Autodesk Inventor part; units mm, degrees
(part 2 of 5)
sketch "Block3" plane through (0, 0, 0) normal (0, 0, 1) x (1, 0, 0)
  line L0 (3.025, -7.2875) -> (16.025, -7.2875)
  line L1 (3.025, -21.2875) -> (16.025, -21.2875)
  line L2 (2.525, -7.7875) -> (2.525, -20.7875)
  line L3 (16.525, -7.7875) -> (16.525, -20.7875)
  arc A0 (3.025, -7.2875) -> (2.525, -7.7875) centre (3.025, -7.7875) ccw
  arc A1 (16.525, -7.7875) -> (16.025, -7.2875) centre (16.025, -7.7875) ccw
  arc A2 (2.525, -20.7875) -> (3.025, -21.2875) centre (3.025, -20.7875) ccw
  arc A3 (16.025, -21.2875) -> (16.525, -20.7875) centre (16.025, -20.7875) ccw
  line L4 (41.125, -7.2875) -> (54.125, -7.2875)
  line L5 (41.125, -21.2875) -> (54.125, -21.2875)
  line L6 (40.625, -7.7875) -> (40.625, -20.7875)
  line L7 (54.625, -7.7875) -> (54.625, -20.7875)
  arc A4 (41.125, -7.2875) -> (40.625, -7.7875) centre (41.125, -7.7875) ccw
  arc A5 (54.625, -7.7875) -> (54.125, -7.2875) centre (54.125, -7.7875) ccw
  arc A6 (40.625, -20.7875) -> (41.125, -21.2875) centre (41.125, -20.7875) ccw
  arc A7 (54.125, -21.2875) -> (54.625, -20.7875) centre (54.125, -20.7875) ccw
  line L8 (60.175, -7.2875) -> (73.175, -7.2875)
  line L9 (60.175, -21.2875) -> (73.175, -21.2875)
  line L10 (59.675, -7.7875) -> (59.675, -20.7875)
  line L11 (73.675, -7.7875) -> (73.675, -20.7875)
  arc A8 (60.175, -7.2875) -> (59.675, -7.7875) centre (60.175, -7.7875) ccw
  arc A9 (73.675, -7.7875) -> (73.175, -7.2875) centre (73.175, -7.7875) ccw
  arc A10 (59.675, -20.7875) -> (60.175, -21.2875) centre (60.175, -20.7875) ccw
  arc A11 (73.175, -21.2875) -> (73.675, -20.7875) centre (73.175, -20.7875) ccw
  line L12 (79.225, -7.2875) -> (92.225, -7.2875)
  line L13 (79.225, -21.2875) -> (92.225, -21.2875)
  line L14 (78.725, -7.7875) -> (78.725, -20.7875)
  line L15 (92.725, -7.7875) -> (92.725, -20.7875)
  arc A12 (79.225, -7.2875) -> (78.725, -7.7875) centre (79.225, -7.7875) ccw
  arc A13 (92.725, -7.7875) -> (92.225, -7.2875) centre (92.225, -7.7875) ccw
  arc A14 (78.725, -20.7875) -> (79.225, -21.2875) centre (79.225, -20.7875) ccw
  arc A15 (92.225, -21.2875) -> (92.725, -20.7875) centre (92.225, -20.7875) ccw
  line L16 (98.275, -7.2875) -> (111.275, -7.2875)
  line L17 (98.275, -21.2875) -> (111.275, -21.2875)
  line L18 (97.775, -7.7875) -> (97.775, -20.7875)
  line L19 (111.775, -7.7875) -> (111.775, -20.7875)
  arc A16 (98.275, -7.2875) -> (97.775, -7.7875) centre (98.275, -7.7875) ccw
  arc A17 (111.775, -7.7875) -> (111.275, -7.2875) centre (111.275, -7.7875) ccw
  arc A18 (97.775, -20.7875) -> (98.275, -21.2875) centre (98.275, -20.7875) ccw
  arc A19 (111.275, -21.2875) -> (111.775, -20.7875) centre (111.275, -20.7875) ccw
  line L20 (126.85, -7.2875) -> (139.85, -7.2875)
  line L21 (126.85, -21.2875) -> (139.85, -21.2875)
  line L22 (126.35, -7.7875) -> (126.35, -20.7875)
  line L23 (140.35, -7.7875) -> (140.35, -20.7875)
  arc A20 (126.85, -7.2875) -> (126.35, -7.7875) centre (126.85, -7.7875) ccw
  arc A21 (140.35, -7.7875) -> (139.85, -7.2875) centre (139.85, -7.7875) ccw
  arc A22 (126.35, -20.7875) -> (126.85, -21.2875) centre (126.85, -20.7875) ccw
  arc A23 (139.85, -21.2875) -> (140.35, -20.7875) centre (139.85, -20.7875) ccw
  line L24 (145.9, -7.2875) -> (158.9, -7.2875)
  line L25 (145.9, -21.2875) -> (158.9, -21.2875)
  line L26 (145.4, -7.7875) -> (145.4, -20.7875)
  line L27 (159.4, -7.7875) -> (159.4, -20.7875)
  arc A24 (145.9, -7.2875) -> (145.4, -7.7875) centre (145.9, -7.7875) ccw
  arc A25 (159.4, -7.7875) -> (158.9, -7.2875) centre (158.9, -7.7875) ccw
  arc A26 (145.4, -20.7875) -> (145.9, -21.2875) centre (145.9, -20.7875) ccw
  arc A27 (158.9, -21.2875) -> (159.4, -20.7875) centre (158.9, -20.7875) ccw
  line L28 (164.95, -7.2875) -> (177.95, -7.2875)
  line L29 (164.95, -21.2875) -> (177.95, -21.2875)
  line L30 (164.45, -7.7875) -> (164.45, -20.7875)
  line L31 (178.45, -7.7875) -> (178.45, -20.7875)
  arc A28 (164.95, -7.2875) -> (164.45, -7.7875) centre (164.95, -7.7875) ccw
  arc A29 (178.45, -7.7875) -> (177.95, -7.2875) centre (177.95, -7.7875) ccw
  arc A30 (164.45, -20.7875) -> (164.95, -21.2875) centre (164.95, -20.7875) ccw
  arc A31 (177.95, -21.2875) -> (178.45, -20.7875) centre (177.95, -20.7875) ccw
  line L32 (184, -7.2875) -> (197, -7.2875)
  line L33 (184, -21.2875) -> (197, -21.2875)
  line L34 (183.5, -7.7875) -> (183.5, -20.7875)
  line L35 (197.5, -7.7875) -> (197.5, -20.7875)
  arc A32 (184, -7.2875) -> (183.5, -7.7875) centre (184, -7.7875) ccw
  arc A33 (197.5, -7.7875) -> (197, -7.2875) centre (197, -7.7875) ccw
  arc A34 (183.5, -20.7875) -> (184, -21.2875) centre (184, -20.7875) ccw
  arc A35 (197, -21.2875) -> (197.5, -20.7875) centre (197, -20.7875) ccw
  line L36 (212.575, -7.2875) -> (225.575, -7.2875)
  line L37 (212.575, -21.2875) -> (225.575, -21.2875)
  line L38 (212.075, -7.7875) -> (212.075, -20.7875)
  line L39 (226.075, -7.7875) -> (226.075, -20.7875)
  arc A36 (212.575, -7.2875) -> (212.075, -7.7875) centre (212.575, -7.7875) ccw
  arc A37 (226.075, -7.7875) -> (225.575, -7.2875) centre (225.575, -7.7875) ccw
  arc A38 (212.075, -20.7875) -> (212.575, -21.2875) centre (212.575, -20.7875) ccw
  arc A39 (225.575, -21.2875) -> (226.075, -20.7875) centre (225.575, -20.7875) ccw
  line L40 (231.625, -7.2875) -> (244.625, -7.2875)
  line L41 (231.625, -21.2875) -> (244.625, -21.2875)
  line L42 (231.125, -7.7875) -> (231.125, -20.7875)
  line L43 (245.125, -7.7875) -> (245.125, -20.7875)
  arc A40 (231.625, -7.2875) -> (231.125, -7.7875) centre (231.625, -7.7875) ccw
  arc A41 (245.125, -7.7875) -> (244.625, -7.2875) centre (244.625, -7.7875) ccw
  arc A42 (231.125, -20.7875) -> (231.625, -21.2875) centre (231.625, -20.7875) ccw
  arc A43 (244.625, -21.2875) -> (245.125, -20.7875) centre (244.625, -20.7875) ccw
  line L44 (250.675, -7.2875) -> (263.675, -7.2875)
  line L45 (250.675, -21.2875) -> (263.675, -21.2875)
  line L46 (250.175, -7.7875) -> (250.175, -20.7875)
  line L47 (264.175, -7.7875) -> (264.175, -20.7875)
  arc A44 (250.675, -7.2875) -> (250.175, -7.7875) centre (250.675, -7.7875) ccw
  arc A45 (264.175, -7.7875) -> (263.675, -7.2875) centre (263.675, -7.7875) ccw
  arc A46 (250.175, -20.7875) -> (250.675, -21.2875) centre (250.675, -20.7875) ccw
  arc A47 (263.675, -21.2875) -> (264.175, -20.7875) centre (263.675, -20.7875) ccw
  line L48 (269.725, -7.2875) -> (282.725, -7.2875)
  line L49 (269.725, -21.2875) -> (282.725, -21.2875)
  line L50 (269.225, -7.7875) -> (269.225, -20.7875)
  line L51 (283.225, -7.7875) -> (283.225, -20.7875)
  arc A48 (269.725, -7.2875) -> (269.225, -7.7875) centre (269.725, -7.7875) ccw
  arc A49 (283.225, -7.7875) -> (282.725, -7.2875) centre (282.725, -7.7875) ccw
  arc A50 (269.225, -20.7875) -> (269.725, -21.2875) centre (269.725, -20.7875) ccw
  arc A51 (282.725, -21.2875) -> (283.225, -20.7875) centre (282.725, -20.7875) ccw
  line L52 (3.025, -31.1) -> (16.025, -31.1)
  line L53 (3.025, -45.1) -> (16.025, -45.1)
  line L54 (2.525, -31.6) -> (2.525, -44.6)
  line L55 (16.525, -31.6) -> (16.525, -44.6)
  arc A52 (3.025, -31.1) -> (2.525, -31.6) centre (3.025, -31.6) ccw
  arc A53 (16.525, -31.6) -> (16.025, -31.1) centre (16.025, -31.6) ccw
  arc A54 (2.525, -44.6) -> (3.025, -45.1) centre (3.025, -44.6) ccw
  arc A55 (16.025, -45.1) -> (16.525, -44.6) centre (16.025, -44.6) ccw
  line L56 (22.075, -31.1) -> (35.075, -31.1)
  line L57 (22.075, -45.1) -> (35.075, -45.1)
  line L58 (21.575, -31.6) -> (21.575, -44.6)
  line L59 (35.575, -31.6) -> (35.575, -44.6)
  arc A56 (22.075, -31.1) -> (21.575, -31.6) centre (22.075, -31.6) ccw
  arc A57 (35.575, -31.6) -> (35.075, -31.1) centre (35.075, -31.6) ccw
  arc A58 (21.575, -44.6) -> (22.075, -45.1) centre (22.075, -44.6) ccw
  arc A59 (35.075, -45.1) -> (35.575, -44.6) centre (35.075, -44.6) ccw
  line L60 (41.125, -31.1) -> (54.125, -31.1)
  line L61 (41.125, -45.1) -> (54.125, -45.1)
  line L62 (40.625, -31.6) -> (40.625, -44.6)
  line L63 (54.625, -31.6) -> (54.625, -44.6)
  arc A60 (41.125, -31.1) -> (40.625, -31.6) centre (41.125, -31.6) ccw
  arc A61 (54.625, -31.6) -> (54.125, -31.1) centre (54.125, -31.6) ccw
  arc A62 (40.625, -44.6) -> (41.125, -45.1) centre (41.125, -44.6) ccw
  arc A63 (54.125, -45.1) -> (54.625, -44.6) centre (54.125, -44.6) ccw
  line L64 (60.175, -31.1) -> (73.175, -31.1)
  line L65 (60.175, -45.1) -> (73.175, -45.1)
  line L66 (59.675, -31.6) -> (59.675, -44.6)
  line L67 (73.675, -31.6) -> (73.675, -44.6)
  arc A64 (60.175, -31.1) -> (59.675, -31.6) centre (60.175, -31.6) ccw
  arc A65 (73.675, -31.6) -> (73.175, -31.1) centre (73.175, -31.6) ccw
  arc A66 (59.675, -44.6) -> (60.175, -45.1) centre (60.175, -44.6) ccw
  arc A67 (73.175, -45.1) -> (73.675, -44.6) centre (73.175, -44.6) ccw
  line L68 (79.225, -31.1) -> (92.225, -31.1)
  line L69 (79.225, -45.1) -> (92.225, -45.1)
  line L70 (78.725, -31.6) -> (78.725, -44.6)
  line L71 (92.725, -31.6) -> (92.725, -44.6)
  arc A68 (79.225, -31.1) -> (78.725, -31.6) centre (79.225, -31.6) ccw
  arc A69 (92.725, -31.6) -> (92.225, -31.1) centre (92.225, -31.6) ccw
  arc A70 (78.725, -44.6) -> (79.225, -45.1) centre (79.225, -44.6) ccw
  arc A71 (92.225, -45.1) -> (92.725, -44.6) centre (92.225, -44.6) ccw
  line L72 (98.275, -31.1) -> (111.275, -31.1)
  line L73 (98.275, -45.1) -> (111.275, -45.1)
  line L74 (97.775, -31.6) -> (97.775, -44.6)
  line L75 (111.775, -31.6) -> (111.775, -44.6)
  arc A72 (98.275, -31.1) -> (97.775, -31.6) centre (98.275, -31.6) ccw
  arc A73 (111.775, -31.6) -> (111.275, -31.1) centre (111.275, -31.6) ccw
  arc A74 (97.775, -44.6) -> (98.275, -45.1) centre (98.275, -44.6) ccw
  arc A75 (111.275, -45.1) -> (111.775, -44.6) centre (111.275, -44.6) ccw
  line L76 (117.325, -31.1) -> (130.325, -31.1)
  line L77 (117.325, -45.1) -> (130.325, -45.1)
  line L78 (116.825, -31.6) -> (116.825, -44.6)
  line L79 (130.825, -31.6) -> (130.825, -44.6)
  arc A76 (117.325, -31.1) -> (116.825, -31.6) centre (117.325, -31.6) ccw
  arc A77 (130.825, -31.6) -> (130.325, -31.1) centre (130.325, -31.6) ccw
  arc A78 (116.825, -44.6) -> (117.325, -45.1) centre (117.325, -44.6) ccw
  arc A79 (130.325, -45.1) -> (130.825, -44.6) centre (130.325, -44.6) ccw
  line L80 (136.375, -31.1) -> (149.375, -31.1)
  line L81 (136.375, -45.1) -> (149.375, -45.1)
  line L82 (135.875, -31.6) -> (135.875, -44.6)
  line L83 (149.875, -31.6) -> (149.875, -44.6)
  arc A80 (136.375, -31.1) -> (135.875, -31.6) centre (136.375, -31.6) ccw
  arc A81 (149.875, -31.6) -> (149.375, -31.1) centre (149.375, -31.6) ccw
  arc A82 (135.875, -44.6) -> (136.375, -45.1) centre (136.375, -44.6) ccw
  arc A83 (149.375, -45.1) -> (149.875, -44.6) centre (149.375, -44.6) ccw
  line L84 (155.425, -31.1) -> (168.425, -31.1)
  line L85 (155.425, -45.1) -> (168.425, -45.1)
  line L86 (154.925, -31.6) -> (154.925, -44.6)
  line L87 (168.925, -31.6) -> (168.925, -44.6)
  arc A84 (155.425, -31.1) -> (154.925, -31.6) centre (155.425, -31.6) ccw
  arc A85 (168.925, -31.6) -> (168.425, -31.1) centre (168.425, -31.6) ccw
  arc A86 (154.925, -44.6) -> (155.425, -45.1) centre (155.425, -44.6) ccw
  arc A87 (168.425, -45.1) -> (168.925, -44.6) centre (168.425, -44.6) ccw
  line L88 (174.475, -31.1) -> (187.475, -31.1)
  line L89 (174.475, -45.1) -> (187.475, -45.1)
  line L90 (173.975, -31.6) -> (173.975, -44.6)
  line L91 (187.975, -31.6) -> (187.975, -44.6)
  arc A88 (174.475, -31.1) -> (173.975, -31.6) centre (174.475, -31.6) ccw
  arc A89 (187.975, -31.6) -> (187.475, -31.1) centre (187.475, -31.6) ccw
  arc A90 (173.975, -44.6) -> (174.475, -45.1) centre (174.475, -44.6) ccw
  arc A91 (187.475, -45.1) -> (187.975, -44.6) centre (187.475, -44.6) ccw
  line L92 (193.525, -31.1) -> (206.525, -31.1)
  line L93 (193.525, -45.1) -> (206.525, -45.1)
  line L94 (193.025, -31.6) -> (193.025, -44.6)
  line L95 (207.025, -31.6) -> (207.025, -44.6)
  arc A92 (193.525, -31.1) -> (193.025, -31.6) centre (193.525, -31.6) ccw
  arc A93 (207.025, -31.6) -> (206.525, -31.1) centre (206.525, -31.6) ccw
  arc A94 (193.025, -44.6) -> (193.525, -45.1) centre (193.525, -44.6) ccw
  arc A95 (206.525, -45.1) -> (207.025, -44.6) centre (206.525, -44.6) ccw
  line L96 (212.575, -31.1) -> (225.575, -31.1)
  line L97 (212.575, -45.1) -> (225.575, -45.1)
  line L98 (212.075, -31.6) -> (212.075, -44.6)
  line L99 (226.075, -31.6) -> (226.075, -44.6)
  arc A96 (212.575, -31.1) -> (212.075, -31.6) centre (212.575, -31.6) ccw
  arc A97 (226.075, -31.6) -> (225.575, -31.1) centre (225.575, -31.6) ccw
  arc A98 (212.075, -44.6) -> (212.575, -45.1) centre (212.575, -44.6) ccw
  arc A99 (225.575, -45.1) -> (226.075, -44.6) centre (225.575, -44.6) ccw
  line L100 (231.625, -31.1) -> (244.625, -31.1)
  line L101 (231.625, -45.1) -> (244.625, -45.1)
  line L102 (231.125, -31.6) -> (231.125, -44.6)
  line L103 (245.125, -31.6) -> (245.125, -44.6)
  arc A100 (231.625, -31.1) -> (231.125, -31.6) centre (231.625, -31.6) ccw
  arc A101 (245.125, -31.6) -> (244.625, -31.1) centre (244.625, -31.6) ccw
  arc A102 (231.125, -44.6) -> (231.625, -45.1) centre (231.625, -44.6) ccw
  arc A103 (244.625, -45.1) -> (245.125, -44.6) centre (244.625, -44.6) ccw
  line L104 (260.2, -31.1) -> (273.2, -31.1)
  line L105 (260.2, -45.1) -> (273.2, -45.1)
  line L106 (259.7, -31.6) -> (259.7, -44.6)
  line L107 (273.7, -31.6) -> (273.7, -44.6)
  arc A104 (260.2, -31.1) -> (259.7, -31.6) centre (260.2, -31.6) ccw
  arc A105 (273.7, -31.6) -> (273.2, -31.1) centre (273.2, -31.6) ccw
  arc A106 (259.7, -44.6) -> (260.2, -45.1) centre (260.2, -44.6) ccw
  arc A107 (273.2, -45.1) -> (273.7, -44.6) centre (273.2, -44.6) ccw
  line L108 (251.762, -32.1) -> (257.762, -32.1)
  line L109 (251.762, -47.1) -> (257.762, -47.1)
  line L110 (251.262, -32.6) -> (251.262, -46.6)
  line L111 (258.262, -32.6) -> (258.262, -46.6)
  arc A108 (251.762, -32.1) -> (251.262, -32.6) centre (251.762, -32.6) ccw
  arc A109 (258.262, -32.6) -> (257.762, -32.1) centre (257.762, -32.6) ccw
  arc A110 (251.262, -46.6) -> (251.762, -47.1) centre (251.762, -46.6) ccw
  arc A111 (257.762, -47.1) -> (258.262, -46.6) centre (257.762, -46.6) ccw
  line L112 (275.638, -32.1) -> (281.638, -32.1)
  line L113 (275.638, -47.1) -> (281.638, -47.1)
  line L114 (275.138, -32.6) -> (275.138, -46.6)
  line L115 (282.138, -32.6) -> (282.138, -46.6)
  arc A112 (275.638, -32.1) -> (275.138, -32.6) centre (275.638, -32.6) ccw
  arc A113 (282.138, -32.6) -> (281.638, -32.1) centre (281.638, -32.6) ccw
  arc A114 (275.138, -46.6) -> (275.638, -47.1) centre (275.638, -46.6) ccw
  arc A115 (281.638, -47.1) -> (282.138, -46.6) centre (281.638, -46.6) ccw
  line L116 (293.5375, -31.1) -> (306.5375, -31.1)
  line L117 (293.5375, -45.1) -> (306.5375, -45.1)
  line L118 (293.0375, -31.6) -> (293.0375, -44.6)
  line L119 (307.0375, -31.6) -> (307.0375, -44.6)
  arc A116 (293.5375, -31.1) -> (293.0375, -31.6) centre (293.5375, -31.6) ccw
  arc A117 (307.0375, -31.6) -> (306.5375, -31.1) centre (306.5375, -31.6) ccw
  arc A118 (293.0375, -44.6) -> (293.5375, -45.1) centre (293.5375, -44.6) ccw
  arc A119 (306.5375, -45.1) -> (307.0375, -44.6) centre (306.5375, -44.6) ccw
  line L120 (312.5875, -31.1) -> (325.5875, -31.1)
  line L121 (312.5875, -45.1) -> (325.5875, -45.1)
  line L122 (312.0875, -31.6) -> (312.0875, -44.6)
  line L123 (326.0875, -31.6) -> (326.0875, -44.6)
  arc A120 (312.5875, -31.1) -> (312.0875, -31.6) centre (312.5875, -31.6) ccw
  arc A121 (326.0875, -31.6) -> (325.5875, -31.1) centre (325.5875, -31.6) ccw
  arc A122 (312.0875, -44.6) -> (312.5875, -45.1) centre (312.5875, -44.6) ccw
  arc A123 (325.5875, -45.1) -> (326.0875, -44.6) centre (325.5875, -44.6) ccw
  line L124 (331.6375, -31.1) -> (344.6375, -31.1)
  line L125 (331.6375, -45.1) -> (344.6375, -45.1)
  line L126 (331.1375, -31.6) -> (331.1375, -44.6)
  line L127 (345.1375, -31.6) -> (345.1375, -44.6)
  arc A124 (331.6375, -31.1) -> (331.1375, -31.6) centre (331.6375, -31.6) ccw
  arc A125 (345.1375, -31.6) -> (344.6375, -31.1) centre (344.6375, -31.6) ccw
  arc A126 (331.1375, -44.6) -> (331.6375, -45.1) centre (331.6375, -44.6) ccw
  arc A127 (344.6375, -45.1) -> (345.1375, -44.6) centre (344.6375, -44.6) ccw
  line L128 (7.7875, -50.15) -> (20.7875, -50.15)
  line L129 (7.7875, -64.15) -> (20.7875, -64.15)
  line L130 (7.2875, -50.65) -> (7.2875, -63.65)
  line L131 (21.2875, -50.65) -> (21.2875, -63.65)
  arc A128 (7.7875, -50.15) -> (7.2875, -50.65) centre (7.7875, -50.65) ccw
  arc A129 (21.2875, -50.65) -> (20.7875, -50.15) centre (20.7875, -50.65) ccw
  arc A130 (7.2875, -63.65) -> (7.7875, -64.15) centre (7.7875, -63.65) ccw
  arc A131 (20.7875, -64.15) -> (21.2875, -63.65) centre (20.7875, -63.65) ccw
  line L132 (31.6, -50.15) -> (44.6, -50.15)
  line L133 (31.6, -64.15) -> (44.6, -64.15)
  line L134 (31.1, -50.65) -> (31.1, -63.65)
  line L135 (45.1, -50.65) -> (45.1, -63.65)
  arc A132 (31.6, -50.15) -> (31.1, -50.65) centre (31.6, -50.65) ccw
  arc A133 (45.1, -50.65) -> (44.6, -50.15) centre (44.6, -50.65) ccw
  arc A134 (31.1, -63.65) -> (31.6, -64.15) centre (31.6, -63.65) ccw
  arc A135 (44.6, -64.15) -> (45.1, -63.65) centre (44.6, -63.65) ccw
  line L136 (50.65, -50.15) -> (63.65, -50.15)
  line L137 (50.65, -64.15) -> (63.65, -64.15)
  line L138 (50.15, -50.65) -> (50.15, -63.65)
  line L139 (64.15, -50.65) -> (64.15, -63.65)
  arc A136 (50.65, -50.15) -> (50.15, -50.65) centre (50.65, -50.65) ccw
  arc A137 (64.15, -50.65) -> (63.65, -50.15) centre (63.65, -50.65) ccw
  arc A138 (50.15, -63.65) -> (50.65, -64.15) centre (50.65, -63.65) ccw
  arc A139 (63.65, -64.15) -> (64.15, -63.65) centre (63.65, -63.65) ccw
  line L140 (69.7, -50.15) -> (82.7, -50.15)
  line L141 (69.7, -64.15) -> (82.7, -64.15)
  line L142 (69.2, -50.65) -> (69.2, -63.65)
  line L143 (83.2, -50.65) -> (83.2, -63.65)
  arc A140 (69.7, -50.15) -> (69.2, -50.65) centre (69.7, -50.65) ccw
  arc A141 (83.2, -50.65) -> (82.7, -50.15) centre (82.7, -50.65) ccw
  arc A142 (69.2, -63.65) -> (69.7, -64.15) centre (69.7, -63.65) ccw
  arc A143 (82.7, -64.15) -> (83.2, -63.65) centre (82.7, -63.65) ccw
  line L144 (88.75, -50.15) -> (101.75, -50.15)
  line L145 (88.75, -64.15) -> (101.75, -64.15)
  line L146 (88.25, -50.65) -> (88.25, -63.65)
  line L147 (102.25, -50.65) -> (102.25, -63.65)
  arc A144 (88.75, -50.15) -> (88.25, -50.65) centre (88.75, -50.65) ccw
  arc A145 (102.25, -50.65) -> (101.75, -50.15) centre (101.75, -50.65) ccw
  arc A146 (88.25, -63.65) -> (88.75, -64.15) centre (88.75, -63.65) ccw
  arc A147 (101.75, -64.15) -> (102.25, -63.65) centre (101.75, -63.65) ccw
  line L148 (107.8, -50.15) -> (120.8, -50.15)
  line L149 (107.8, -64.15) -> (120.8, -64.15)
  line L150 (107.3, -50.65) -> (107.3, -63.65)
  line L151 (121.3, -50.65) -> (121.3, -63.65)
  arc A148 (107.8, -50.15) -> (107.3, -50.65) centre (107.8, -50.65) ccw
  arc A149 (121.3, -50.65) -> (120.8, -50.15) centre (120.8, -50.65) ccw
  arc A150 (107.3, -63.65) -> (107.8, -64.15) centre (107.8, -63.65) ccw
  arc A151 (120.8, -64.15) -> (121.3, -63.65) centre (120.8, -63.65) ccw
  line L152 (126.85, -50.15) -> (139.85, -50.15)
  line L153 (126.85, -64.15) -> (139.85, -64.15)
  line L154 (126.35, -50.65) -> (126.35, -63.65)
  line L155 (140.35, -50.65) -> (140.35, -63.65)
  arc A152 (126.85, -50.15) -> (126.35, -50.65) centre (126.85, -50.65) ccw
  arc A153 (140.35, -50.65) -> (139.85, -50.15) centre (139.85, -50.65) ccw
  arc A154 (126.35, -63.65) -> (126.85, -64.15) centre (126.85, -63.65) ccw
  arc A155 (139.85, -64.15) -> (140.35, -63.65) centre (139.85, -63.65) ccw
  line L156 (145.9, -50.15) -> (158.9, -50.15)
  line L157 (145.9, -64.15) -> (158.9, -64.15)
  line L158 (145.4, -50.65) -> (145.4, -63.65)
  line L159 (159.4, -50.65) -> (159.4, -63.65)
  arc A156 (145.9, -50.15) -> (145.4, -50.65) centre (145.9, -50.65) ccw
  arc A157 (159.4, -50.65) -> (158.9, -50.15) centre (158.9, -50.65) ccw
  arc A158 (145.4, -63.65) -> (145.9, -64.15) centre (145.9, -63.65) ccw
  arc A159 (158.9, -64.15) -> (159.4, -63.65) centre (158.9, -63.65) ccw
  line L160 (164.95, -50.15) -> (177.95, -50.15)
  line L161 (164.95, -64.15) -> (177.95, -64.15)
  line L162 (164.45, -50.65) -> (164.45, -63.65)
  line L163 (178.45, -50.65) -> (178.45, -63.65)
  arc A160 (164.95, -50.15) -> (164.45, -50.65) centre (164.95, -50.65) ccw
  arc A161 (178.45, -50.65) -> (177.95, -50.15) centre (177.95, -50.65) ccw
  arc A162 (164.45, -63.65) -> (164.95, -64.15) centre (164.95, -63.65) ccw
  arc A163 (177.95, -64.15) -> (178.45, -63.65) centre (177.95, -63.65) ccw
  line L164 (184, -50.15) -> (197, -50.15)
  line L165 (184, -64.15) -> (197, -64.15)
  line L166 (183.5, -50.65) -> (183.5, -63.65)
  line L167 (197.5, -50.65) -> (197.5, -63.65)
  arc A164 (184, -50.15) -> (183.5, -50.65) centre (184, -50.65) ccw
  arc A165 (197.5, -50.65) -> (197, -50.15) centre (197, -50.65) ccw
  arc A166 (183.5, -63.65) -> (184, -64.15) centre (184, -63.65) ccw
  arc A167 (197, -64.15) -> (197.5, -63.65) centre (197, -63.65) ccw
  line L168 (203.05, -50.15) -> (216.05, -50.15)
  line L169 (203.05, -64.15) -> (216.05, -64.15)
  line L170 (202.55, -50.65) -> (202.55, -63.65)
  line L171 (216.55, -50.65) -> (216.55, -63.65)
  arc A168 (203.05, -50.15) -> (202.55, -50.65) centre (203.05, -50.65) ccw
  arc A169 (216.55, -50.65) -> (216.05, -50.15) centre (216.05, -50.65) ccw
  arc A170 (202.55, -63.65) -> (203.05, -64.15) centre (203.05, -63.65) ccw
  arc A171 (216.05, -64.15) -> (216.55, -63.65) centre (216.05, -63.65) ccw
  line L172 (222.1, -50.15) -> (235.1, -50.15)
  line L173 (222.1, -64.15) -> (235.1, -64.15)
  line L174 (221.6, -50.65) -> (221.6, -63.65)
  line L175 (235.6, -50.65) -> (235.6, -63.65)
  arc A172 (222.1, -50.15) -> (221.6, -50.65) centre (222.1, -50.65) ccw
  arc A173 (235.6, -50.65) -> (235.1, -50.15) centre (235.1, -50.65) ccw
  arc A174 (221.6, -63.65) -> (222.1, -64.15) centre (222.1, -63.65) ccw
  arc A175 (235.1, -64.15) -> (235.6, -63.65) centre (235.1, -63.65) ccw
  line L176 (241.15, -50.15) -> (254.15, -50.15)
  line L177 (241.15, -64.15) -> (254.15, -64.15)
  line L178 (240.65, -50.65) -> (240.65, -63.65)
  line L179 (254.65, -50.65) -> (254.65, -63.65)
  arc A176 (241.15, -50.15) -> (240.65, -50.65) centre (241.15, -50.65) ccw
  arc A177 (254.65, -50.65) -> (254.15, -50.15) centre (254.15, -50.65) ccw
  arc A178 (240.65, -63.65) -> (241.15, -64.15) centre (241.15, -63.65) ccw
  arc A179 (254.15, -64.15) -> (254.65, -63.65) centre (254.15, -63.65) ccw
  line L180 (264.9625, -50.15) -> (277.9625, -50.15)
  line L181 (264.9625, -64.15) -> (277.9625, -64.15)
  line L182 (264.4625, -50.65) -> (264.4625, -63.65)
  line L183 (278.4625, -50.65) -> (278.4625, -63.65)
  arc A180 (264.9625, -50.15) -> (264.4625, -50.65) centre (264.9625, -50.65) ccw
  arc A181 (278.4625, -50.65) -> (277.9625, -50.15) centre (277.9625, -50.65) ccw
  arc A182 (264.4625, -63.65) -> (264.9625, -64.15) centre (264.9625, -63.65) ccw
  arc A183 (277.9625, -64.15) -> (278.4625, -63.65) centre (277.9625, -63.65) ccw
  line L184 (293.5375, -50.15) -> (306.5375, -50.15)
  line L185 (293.5375, -64.15) -> (306.5375, -64.15)
  line L186 (293.0375, -50.65) -> (293.0375, -63.65)
  line L187 (307.0375, -50.65) -> (307.0375, -63.65)
  arc A184 (293.5375, -50.15) -> (293.0375, -50.65) centre (293.5375, -50.65) ccw
  arc A185 (307.0375, -50.65) -> (306.5375, -50.15) centre (306.5375, -50.65) ccw
  arc A186 (293.0375, -63.65) -> (293.5375, -64.15) centre (293.5375, -63.65) ccw
  arc A187 (306.5375, -64.15) -> (307.0375, -63.65) centre (306.5375, -63.65) ccw
  line L188 (312.5875, -50.15) -> (325.5875, -50.15)
  line L189 (312.5875, -64.15) -> (325.5875, -64.15)
  line L190 (312.0875, -50.65) -> (312.0875, -63.65)
  line L191 (326.0875, -50.65) -> (326.0875, -63.65)
  arc A188 (312.5875, -50.15) -> (312.0875, -50.65) centre (312.5875, -50.65) ccw
  arc A189 (326.0875, -50.65) -> (325.5875, -50.15) centre (325.5875, -50.65) ccw
  arc A190 (312.0875, -63.65) -> (312.5875, -64.15) centre (312.5875, -63.65) ccw
  arc A191 (325.5875, -64.15) -> (326.0875, -63.65) centre (325.5875, -63.65) ccw
  line L192 (331.6375, -50.15) -> (344.6375, -50.15)
  line L193 (331.6375, -64.15) -> (344.6375, -64.15)
  line L194 (331.1375, -50.65) -> (331.1375, -63.65)
  line L195 (345.1375, -50.65) -> (345.1375, -63.65)
  arc A192 (331.6375, -50.15) -> (331.1375, -50.65) centre (331.6375, -50.65) ccw
  arc A193 (345.1375, -50.65) -> (344.6375, -50.15) centre (344.6375, -50.65) ccw
  arc A194 (331.1375, -63.65) -> (331.6375, -64.15) centre (331.6375, -63.65) ccw
  arc A195 (344.6375, -64.15) -> (345.1375, -63.65) centre (344.6375, -63.65) ccw
  line L196 (10.1687, -69.2) -> (23.1687, -69.2)
  line L197 (10.1687, -83.2) -> (23.1687, -83.2)
  line L198 (9.6687, -69.7) -> (9.6687, -82.7)
  line L199 (23.6687, -69.7) -> (23.6687, -82.7)
  arc A196 (10.1687, -69.2) -> (9.6687, -69.7) centre (10.1687, -69.7) ccw
  arc A197 (23.6687, -69.7) -> (23.1687, -69.2) centre (23.1687, -69.7) ccw
  arc A198 (9.6687, -82.7) -> (10.1687, -83.2) centre (10.1687, -82.7) ccw
  arc A199 (23.1687, -83.2) -> (23.6687, -82.7) centre (23.1687, -82.7) ccw
  line L200 (36.3625, -69.2) -> (49.3625, -69.2)
  line L201 (36.3625, -83.2) -> (49.3625, -83.2)
  line L202 (35.8625, -69.7) -> (35.8625, -82.7)
  line L203 (49.8625, -69.7) -> (49.8625, -82.7)
  arc A200 (36.3625, -69.2) -> (35.8625, -69.7) centre (36.3625, -69.7) ccw
  arc A201 (49.8625, -69.7) -> (49.3625, -69.2) centre (49.3625, -69.7) ccw
  arc A202 (35.8625, -82.7) -> (36.3625, -83.2) centre (36.3625, -82.7) ccw
  arc A203 (49.3625, -83.2) -> (49.8625, -82.7) centre (49.3625, -82.7) ccw
  line L204 (55.4125, -69.2) -> (68.4125, -69.2)
  line L205 (55.4125, -83.2) -> (68.4125, -83.2)
  line L206 (54.9125, -69.7) -> (54.9125, -82.7)
  line L207 (68.9125, -69.7) -> (68.9125, -82.7)
  arc A204 (55.4125, -69.2) -> (54.9125, -69.7) centre (55.4125, -69.7) ccw
  arc A205 (68.9125, -69.7) -> (68.4125, -69.2) centre (68.4125, -69.7) ccw
  arc A206 (54.9125, -82.7) -> (55.4125, -83.2) centre (55.4125, -82.7) ccw
  arc A207 (68.4125, -83.2) -> (68.9125, -82.7) centre (68.4125, -82.7) ccw
  line L208 (74.4625, -69.2) -> (87.4625, -69.2)
  line L209 (74.4625, -83.2) -> (87.4625, -83.2)
  line L210 (73.9625, -69.7) -> (73.9625, -82.7)
  line L211 (87.9625, -69.7) -> (87.9625, -82.7)
  arc A208 (74.4625, -69.2) -> (73.9625, -69.7) centre (74.4625, -69.7) ccw
  arc A209 (87.9625, -69.7) -> (87.4625, -69.2) centre (87.4625, -69.7) ccw
  arc A210 (73.9625, -82.7) -> (74.4625, -83.2) centre (74.4625, -82.7) ccw
  arc A211 (87.4625, -83.2) -> (87.9625, -82.7) centre (87.4625, -82.7) ccw
  line L212 (93.5125, -69.2) -> (106.5125, -69.2)
  line L213 (93.5125, -83.2) -> (106.5125, -83.2)
  line L214 (93.0125, -69.7) -> (93.0125, -82.7)
  line L215 (107.0125, -69.7) -> (107.0125, -82.7)
  arc A212 (93.5125, -69.2) -> (93.0125, -69.7) centre (93.5125, -69.7) ccw
  arc A213 (107.0125, -69.7) -> (106.5125, -69.2) centre (106.5125, -69.7) ccw
  arc A214 (93.0125, -82.7) -> (93.5125, -83.2) centre (93.5125, -82.7) ccw
  arc A215 (106.5125, -83.2) -> (107.0125, -82.7) centre (106.5125, -82.7) ccw
  line L216 (112.5625, -69.2) -> (125.5625, -69.2)
  line L217 (112.5625, -83.2) -> (125.5625, -83.2)
  line L218 (112.0625, -69.7) -> (112.0625, -82.7)
  line L219 (126.0625, -69.7) -> (126.0625, -82.7)
  arc A216 (112.5625, -69.2) -> (112.0625, -69.7) centre (112.5625, -69.7) ccw
  arc A217 (126.0625, -69.7) -> (125.5625, -69.2) centre (125.5625, -69.7) ccw
  arc A218 (112.0625, -82.7) -> (112.5625, -83.2) centre (112.5625, -82.7) ccw
  arc A219 (125.5625, -83.2) -> (126.0625, -82.7) centre (125.5625, -82.7) ccw
  line L220 (131.6125, -69.2) -> (144.6125, -69.2)
  line L221 (131.6125, -83.2) -> (144.6125, -83.2)
  line L222 (131.1125, -69.7) -> (131.1125, -82.7)
  line L223 (145.1125, -69.7) -> (145.1125, -82.7)
  arc A220 (131.6125, -69.2) -> (131.1125, -69.7) centre (131.6125, -69.7) ccw
  arc A221 (145.1125, -69.7) -> (144.6125, -69.2) centre (144.6125, -69.7) ccw
  arc A222 (131.1125, -82.7) -> (131.6125, -83.2) centre (131.6125, -82.7) ccw
  arc A223 (144.6125, -83.2) -> (145.1125, -82.7) centre (144.6125, -82.7) ccw
  line L224 (150.6625, -69.2) -> (163.6625, -69.2)
  line L225 (150.6625, -83.2) -> (163.6625, -83.2)
  line L226 (150.1625, -69.7) -> (150.1625, -82.7)
  line L227 (164.1625, -69.7) -> (164.1625, -82.7)
  arc A224 (150.6625, -69.2) -> (150.1625, -69.7) centre (150.6625, -69.7) ccw
  arc A225 (164.1625, -69.7) -> (163.6625, -69.2) centre (163.6625, -69.7) ccw
  arc A226 (150.1625, -82.7) -> (150.6625, -83.2) centre (150.6625, -82.7) ccw
  arc A227 (163.6625, -83.2) -> (164.1625, -82.7) centre (163.6625, -82.7) ccw
  line L228 (169.7125, -69.2) -> (182.7125, -69.2)
  line L229 (169.7125, -83.2) -> (182.7125, -83.2)
  line L230 (169.2125, -69.7) -> (169.2125, -82.7)
  line L231 (183.2125, -69.7) -> (183.2125, -82.7)
  arc A228 (169.7125, -69.2) -> (169.2125, -69.7) centre (169.7125, -69.7) ccw
  arc A229 (183.2125, -69.7) -> (182.7125, -69.2) centre (182.7125, -69.7) ccw
  arc A230 (169.2125, -82.7) -> (169.7125, -83.2) centre (169.7125, -82.7) ccw
  arc A231 (182.7125, -83.2) -> (183.2125, -82.7) centre (182.7125, -82.7) ccw
  line L232 (188.7625, -69.2) -> (201.7625, -69.2)
  line L233 (188.7625, -83.2) -> (201.7625, -83.2)
  line L234 (188.2625, -69.7) -> (188.2625, -82.7)
  line L235 (202.2625, -69.7) -> (202.2625, -82.7)
  arc A232 (188.7625, -69.2) -> (188.2625, -69.7) centre (188.7625, -69.7) ccw
  arc A233 (202.2625, -69.7) -> (201.7625, -69.2) centre (201.7625, -69.7) ccw
  arc A234 (188.2625, -82.7) -> (188.7625, -83.2) centre (188.7625, -82.7) ccw
  arc A235 (201.7625, -83.2) -> (202.2625, -82.7) centre (201.7625, -82.7) ccw
  line L236 (207.8125, -69.2) -> (220.8125, -69.2)
  line L237 (207.8125, -83.2) -> (220.8125, -83.2)
  line L238 (207.3125, -69.7) -> (207.3125, -82.7)
  line L239 (221.3125, -69.7) -> (221.3125, -82.7)
  arc A236 (207.8125, -69.2) -> (207.3125, -69.7) centre (207.8125, -69.7) ccw
  arc A237 (221.3125, -69.7) -> (220.8125, -69.2) centre (220.8125, -69.7) ccw
  arc A238 (207.3125, -82.7) -> (207.8125, -83.2) centre (207.8125, -82.7) ccw
  arc A239 (220.8125, -83.2) -> (221.3125, -82.7) centre (220.8125, -82.7) ccw
  line L240 (226.8625, -69.2) -> (239.8625, -69.2)
  line L241 (226.8625, -83.2) -> (239.8625, -83.2)
  line L242 (226.3625, -69.7) -> (226.3625, -82.7)
  line L243 (240.3625, -69.7) -> (240.3625, -82.7)
  arc A240 (226.8625, -69.2) -> (226.3625, -69.7) centre (226.8625, -69.7) ccw
  arc A241 (240.3625, -69.7) -> (239.8625, -69.2) centre (239.8625, -69.7) ccw
  arc A242 (226.3625, -82.7) -> (226.8625, -83.2) centre (226.8625, -82.7) ccw
  arc A243 (239.8625, -83.2) -> (240.3625, -82.7) centre (239.8625, -82.7) ccw
  line L244 (257.8188, -69.2) -> (270.8188, -69.2)
  line L245 (257.8188, -83.2) -> (270.8188, -83.2)
  line L246 (257.3188, -69.7) -> (257.3188, -82.7)
  line L247 (271.3188, -69.7) -> (271.3188, -82.7)
  arc A244 (257.8188, -69.2) -> (257.3188, -69.7) centre (257.8188, -69.7) ccw
  arc A245 (271.3188, -69.7) -> (270.8188, -69.2) centre (270.8188, -69.7) ccw
  arc A246 (257.3188, -82.7) -> (257.8188, -83.2) centre (257.8188, -82.7) ccw
  arc A247 (270.8188, -83.2) -> (271.3188, -82.7) centre (270.8188, -82.7) ccw
  line L248 (249.3808, -70.2) -> (255.3808, -70.2)
  line L249 (249.3808, -85.2) -> (255.3808, -85.2)
  line L250 (248.8808, -70.7) -> (248.8808, -84.7)
  line L251 (255.8808, -70.7) -> (255.8808, -84.7)
  arc A248 (249.3808, -70.2) -> (248.8808, -70.7) centre (249.3808, -70.7) ccw
  arc A249 (255.8808, -70.7) -> (255.3808, -70.2) centre (255.3808, -70.7) ccw
  arc A250 (248.8808, -84.7) -> (249.3808, -85.2) centre (249.3808, -84.7) ccw
  arc A251 (255.3808, -85.2) -> (255.8808, -84.7) centre (255.3808, -84.7) ccw
  line L252 (273.2568, -70.2) -> (279.2568, -70.2)
  line L253 (273.2568, -85.2) -> (279.2568, -85.2)
  line L254 (272.7568, -70.7) -> (272.7568, -84.7)
  line L255 (279.7568, -70.7) -> (279.7568, -84.7)
  arc A252 (273.2568, -70.2) -> (272.7568, -70.7) centre (273.2568, -70.7) ccw
  arc A253 (279.7568, -70.7) -> (279.2568, -70.2) centre (279.2568, -70.7) ccw
  arc A254 (272.7568, -84.7) -> (273.2568, -85.2) centre (273.2568, -84.7) ccw
  arc A255 (279.2568, -85.2) -> (279.7568, -84.7) centre (279.2568, -84.7) ccw
  line L256 (14.9313, -88.25) -> (27.9312, -88.25)
  line L257 (14.9313, -102.25) -> (27.9312, -102.25)
  line L258 (14.4313, -88.75) -> (14.4313, -101.75)
  line L259 (28.4313, -88.75) -> (28.4313, -101.75)
  arc A256 (14.9313, -88.25) -> (14.4313, -88.75) centre (14.9313, -88.75) ccw
  arc A257 (28.4313, -88.75) -> (27.9312, -88.25) centre (27.9312, -88.75) ccw
  arc A258 (14.4313, -101.75) -> (14.9313, -102.25) centre (14.9313, -101.75) ccw
  arc A259 (27.9312, -102.25) -> (28.4313, -101.75) centre (27.9312, -101.75) ccw
  line L260 (6.4933, -89.25) -> (12.4932, -89.25)
  line L261 (6.4933, -104.25) -> (12.4932, -104.25)
  line L262 (5.9932, -89.75) -> (5.9932, -103.75)
  line L263 (12.9932, -89.75) -> (12.9932, -103.75)
  arc A260 (6.4933, -89.25) -> (5.9932, -89.75) centre (6.4933, -89.75) ccw
  arc A261 (12.9932, -89.75) -> (12.4932, -89.25) centre (12.4932, -89.75) ccw
  arc A262 (5.9932, -103.75) -> (6.4933, -104.25) centre (6.4933, -103.75) ccw
  arc A263 (12.4932, -104.25) -> (12.9932, -103.75) centre (12.4932, -103.75) ccw
  line L264 (30.3693, -89.25) -> (36.3693, -89.25)
  line L265 (30.3693, -104.25) -> (36.3693, -104.25)
  line L266 (29.8693, -89.75) -> (29.8693, -103.75)
  line L267 (36.8693, -89.75) -> (36.8693, -103.75)
  arc A264 (30.3693, -89.25) -> (29.8693, -89.75) centre (30.3693, -89.75) ccw
  arc A265 (36.8693, -89.75) -> (36.3693, -89.25) centre (36.3693, -89.75) ccw
  arc A266 (29.8693, -103.75) -> (30.3693, -104.25) centre (30.3693, -103.75) ccw
  arc A267 (36.3693, -104.25) -> (36.8693, -103.75) centre (36.3693, -103.75) ccw
  line L268 (45.8875, -88.25) -> (58.8875, -88.25)
  line L269 (45.8875, -102.25) -> (58.8875, -102.25)
  line L270 (45.3875, -88.75) -> (45.3875, -101.75)
  line L271 (59.3875, -88.75) -> (59.3875, -101.75)
  arc A268 (45.8875, -88.25) -> (45.3875, -88.75) centre (45.8875, -88.75) ccw
  arc A269 (59.3875, -88.75) -> (58.8875, -88.25) centre (58.8875, -88.75) ccw
  arc A270 (45.3875, -101.75) -> (45.8875, -102.25) centre (45.8875, -101.75) ccw
  arc A271 (58.8875, -102.25) -> (59.3875, -101.75) centre (58.8875, -101.75) ccw
  line L272 (64.9375, -88.25) -> (77.9375, -88.25)
  line L273 (64.9375, -102.25) -> (77.9375, -102.25)
  line L274 (64.4375, -88.75) -> (64.4375, -101.75)
  line L275 (78.4375, -88.75) -> (78.4375, -101.75)
  arc A272 (64.9375, -88.25) -> (64.4375, -88.75) centre (64.9375, -88.75) ccw
  arc A273 (78.4375, -88.75) -> (77.9375, -88.25) centre (77.9375, -88.75) ccw
  arc A274 (64.4375, -101.75) -> (64.9375, -102.25) centre (64.9375, -101.75) ccw
  arc A275 (77.9375, -102.25) -> (78.4375, -101.75) centre (77.9375, -101.75) ccw
  line L276 (83.9875, -88.25) -> (96.9875, -88.25)
  line L277 (83.9875, -102.25) -> (96.9875, -102.25)
  line L278 (83.4875, -88.75) -> (83.4875, -101.75)
  line L279 (97.4875, -88.75) -> (97.4875, -101.75)
  arc A276 (83.9875, -88.25) -> (83.4875, -88.75) centre (83.9875, -88.75) ccw
  arc A277 (97.4875, -88.75) -> (96.9875, -88.25) centre (96.9875, -88.75) ccw
  arc A278 (83.4875, -101.75) -> (83.9875, -102.25) centre (83.9875, -101.75) ccw
  arc A279 (96.9875, -102.25) -> (97.4875, -101.75) centre (96.9875, -101.75) ccw
  line L280 (103.0375, -88.25) -> (116.0375, -88.25)
  line L281 (103.0375, -102.25) -> (116.0375, -102.25)
  line L282 (102.5375, -88.75) -> (102.5375, -101.75)
  line L283 (116.5375, -88.75) -> (116.5375, -101.75)
  arc A280 (103.0375, -88.25) -> (102.5375, -88.75) centre (103.0375, -88.75) ccw
  arc A281 (116.5375, -88.75) -> (116.0375, -88.25) centre (116.0375, -88.75) ccw
  arc A282 (102.5375, -101.75) -> (103.0375, -102.25) centre (103.0375, -101.75) ccw
  arc A283 (116.0375, -102.25) -> (116.5375, -101.75) centre (116.0375, -101.75) ccw
  line L284 (122.0875, -88.25) -> (135.0875, -88.25)
  line L285 (122.0875, -102.25) -> (135.0875, -102.25)
  line L286 (121.5875, -88.75) -> (121.5875, -101.75)
  line L287 (135.5875, -88.75) -> (135.5875, -101.75)
  arc A284 (122.0875, -88.25) -> (121.5875, -88.75) centre (122.0875, -88.75) ccw
  arc A285 (135.5875, -88.75) -> (135.0875, -88.25) centre (135.0875, -88.75) ccw
  arc A286 (121.5875, -101.75) -> (122.0875, -102.25) centre (122.0875, -101.75) ccw
  arc A287 (135.0875, -102.25) -> (135.5875, -101.75) centre (135.0875, -101.75) ccw
  line L288 (141.1375, -88.25) -> (154.1375, -88.25)
  line L289 (141.1375, -102.25) -> (154.1375, -102.25)
  line L290 (140.6375, -88.75) -> (140.6375, -101.75)
  line L291 (154.6375, -88.75) -> (154.6375, -101.75)
  arc A288 (141.1375, -88.25) -> (140.6375, -88.75) centre (141.1375, -88.75) ccw
  arc A289 (154.6375, -88.75) -> (154.1375, -88.25) centre (154.1375, -88.75) ccw
  arc A290 (140.6375, -101.75) -> (141.1375, -102.25) centre (141.1375, -101.75) ccw
  arc A291 (154.1375, -102.25) -> (154.6375, -101.75) centre (154.1375, -101.75) ccw
  line L292 (160.1875, -88.25) -> (173.1875, -88.25)
  line L293 (160.1875, -102.25) -> (173.1875, -102.25)
  line L294 (159.6875, -88.75) -> (159.6875, -101.75)
  line L295 (173.6875, -88.75) -> (173.6875, -101.75)
  arc A292 (160.1875, -88.25) -> (159.6875, -88.75) centre (160.1875, -88.75) ccw
  arc A293 (173.6875, -88.75) -> (173.1875, -88.25) centre (173.1875, -88.75) ccw
  arc A294 (159.6875, -101.75) -> (160.1875, -102.25) centre (160.1875, -101.75) ccw
  arc A295 (173.1875, -102.25) -> (173.6875, -101.75) centre (173.1875, -101.75) ccw
  line L296 (179.2375, -88.25) -> (192.2375, -88.25)
  line L297 (179.2375, -102.25) -> (192.2375, -102.25)
  line L298 (178.7375, -88.75) -> (178.7375, -101.75)
  line L299 (192.7375, -88.75) -> (192.7375, -101.75)
  arc A296 (179.2375, -88.25) -> (178.7375, -88.75) centre (179.2375, -88.75) ccw
  arc A297 (192.7375, -88.75) -> (192.2375, -88.25) centre (192.2375, -88.75) ccw
  arc A298 (178.7375, -101.75) -> (179.2375, -102.25) centre (179.2375, -101.75) ccw
  arc A299 (192.2375, -102.25) -> (192.7375, -101.75) centre (192.2375, -101.75) ccw
  line L300 (198.2875, -88.25) -> (211.2875, -88.25)
  line L301 (198.2875, -102.25) -> (211.2875, -102.25)
  line L302 (197.7875, -88.75) -> (197.7875, -101.75)
  line L303 (211.7875, -88.75) -> (211.7875, -101.75)
  arc A300 (198.2875, -88.25) -> (197.7875, -88.75) centre (198.2875, -88.75) ccw
  arc A301 (211.7875, -88.75) -> (211.2875, -88.25) centre (211.2875, -88.75) ccw
  arc A302 (197.7875, -101.75) -> (198.2875, -102.25) centre (198.2875, -101.75) ccw
  arc A303 (211.2875, -102.25) -> (211.7875, -101.75) centre (211.2875, -101.75) ccw
  line L304 (217.3375, -88.25) -> (230.3375, -88.25)
  line L305 (217.3375, -102.25) -> (230.3375, -102.25)
  line L306 (216.8375, -88.75) -> (216.8375, -101.75)
  line L307 (230.8375, -88.75) -> (230.8375, -101.75)
  arc A304 (217.3375, -88.25) -> (216.8375, -88.75) centre (217.3375, -88.75) ccw
  arc A305 (230.8375, -88.75) -> (230.3375, -88.25) centre (230.3375, -88.75) ccw
  arc A306 (216.8375, -101.75) -> (217.3375, -102.25) centre (217.3375, -101.75) ccw
  arc A307 (230.3375, -102.25) -> (230.8375, -101.75) centre (230.3375, -101.75) ccw
  line L308 (253.0563, -88.25) -> (266.0562, -88.25)
  line L309 (253.0563, -102.25) -> (266.0562, -102.25)
  line L310 (252.5563, -88.75) -> (252.5563, -101.75)
  line L311 (266.5562, -88.75) -> (266.5562, -101.75)
  arc A308 (253.0563, -88.25) -> (252.5563, -88.75) centre (253.0563, -88.75) ccw
  arc A309 (266.5562, -88.75) -> (266.0562, -88.25) centre (266.0562, -88.75) ccw
  arc A310 (252.5563, -101.75) -> (253.0563, -102.25) centre (253.0563, -101.75) ccw
  arc A311 (266.0562, -102.25) -> (266.5562, -101.75) centre (266.0562, -101.75) ccw
  line L312 (244.6183, -89.25) -> (250.6182, -89.25)
  line L313 (244.6183, -104.25) -> (250.6182, -104.25)
  line L314 (244.1182, -89.75) -> (244.1182, -103.75)
  line L315 (251.1182, -89.75) -> (251.1182, -103.75)
  arc A312 (244.6183, -89.25) -> (244.1182, -89.75) centre (244.6183, -89.75) ccw
  arc A313 (251.1182, -89.75) -> (250.6182, -89.25) centre (250.6182, -89.75) ccw
  arc A314 (244.1182, -103.75) -> (244.6183, -104.25) centre (244.6183, -103.75) ccw
  arc A315 (250.6182, -104.25) -> (251.1182, -103.75) centre (250.6182, -103.75) ccw
  line L316 (268.4943, -89.25) -> (274.4943, -89.25)
  line L317 (268.4943, -104.25) -> (274.4943, -104.25)
  line L318 (267.9943, -89.75) -> (267.9943, -103.75)
  line L319 (274.9943, -89.75) -> (274.9943, -103.75)
  arc A316 (268.4943, -89.25) -> (267.9943, -89.75) centre (268.4943, -89.75) ccw
  arc A317 (274.9943, -89.75) -> (274.4943, -89.25) centre (274.4943, -89.75) ccw
  arc A318 (267.9943, -103.75) -> (268.4943, -104.25) centre (268.4943, -103.75) ccw
  arc A319 (274.4943, -104.25) -> (274.9943, -103.75) centre (274.4943, -103.75) ccw
  line L320 (312.5875, -88.25) -> (325.5875, -88.25)
  line L321 (312.5875, -102.25) -> (325.5875, -102.25)
  line L322 (312.0875, -88.75) -> (312.0875, -101.75)
  line L323 (326.0875, -88.75) -> (326.0875, -101.75)
  arc A320 (312.5875, -88.25) -> (312.0875, -88.75) centre (312.5875, -88.75) ccw
  arc A321 (326.0875, -88.75) -> (325.5875, -88.25) centre (325.5875, -88.75) ccw
  arc A322 (312.0875, -101.75) -> (312.5875, -102.25) centre (312.5875, -101.75) ccw
  arc A323 (325.5875, -102.25) -> (326.0875, -101.75) centre (325.5875, -101.75) ccw
  line L324 (5.4062, -107.3) -> (18.4062, -107.3)
  line L325 (5.4062, -121.3) -> (18.4062, -121.3)
  line L326 (4.9062, -107.8) -> (4.9062, -120.8)
  line L327 (18.9062, -107.8) -> (18.9062, -120.8)
  arc A324 (5.4062, -107.3) -> (4.9062, -107.8) centre (5.4062, -107.8) ccw
  arc A325 (18.9062, -107.8) -> (18.4062, -107.3) centre (18.4062, -107.8) ccw
  arc A326 (4.9062, -120.8) -> (5.4062, -121.3) centre (5.4062, -120.8) ccw
  arc A327 (18.4062, -121.3) -> (18.9062, -120.8) centre (18.4062, -120.8) ccw
  line L328 (29.2188, -107.3) -> (42.2188, -107.3)
  line L329 (29.2188, -121.3) -> (42.2188, -121.3)
  line L330 (28.7188, -107.8) -> (28.7188, -120.8)
  line L331 (42.7188, -107.8) -> (42.7188, -120.8)
  arc A328 (29.2188, -107.3) -> (28.7188, -107.8) centre (29.2188, -107.8) ccw
  arc A329 (42.7188, -107.8) -> (42.2188, -107.3) centre (42.2188, -107.8) ccw
  arc A330 (28.7188, -120.8) -> (29.2188, -121.3) centre (29.2188, -120.8) ccw
  arc A331 (42.2188, -121.3) -> (42.7188, -120.8) centre (42.2188, -120.8) ccw
  line L332 (53.0313, -107.3) -> (66.0312, -107.3)
  line L333 (53.0313, -121.3) -> (66.0312, -121.3)
  line L334 (52.5313, -107.8) -> (52.5313, -120.8)
  line L335 (66.5312, -107.8) -> (66.5312, -120.8)
  arc A332 (53.0313, -107.3) -> (52.5313, -107.8) centre (53.0313, -107.8) ccw
  arc A333 (66.5312, -107.8) -> (66.0312, -107.3) centre (66.0312, -107.8) ccw
  arc A334 (52.5313, -120.8) -> (53.0313, -121.3) centre (53.0313, -120.8) ccw
  arc A335 (66.0312, -121.3) -> (66.5312, -120.8) centre (66.0312, -120.8) ccw
  line L336 (124.4688, -107.3) -> (137.4688, -107.3)
  line L337 (124.4688, -121.3) -> (137.4688, -121.3)
  line L338 (123.9688, -107.8) -> (123.9688, -120.8)
  line L339 (137.9688, -107.8) -> (137.9688, -120.8)
  arc A336 (124.4688, -107.3) -> (123.9688, -107.8) centre (124.4688, -107.8) ccw
  arc A337 (137.9688, -107.8) -> (137.4688, -107.3) centre (137.4688, -107.8) ccw
  arc A338 (123.9688, -120.8) -> (124.4688, -121.3) centre (124.4688, -120.8) ccw
  arc A339 (137.4688, -121.3) -> (137.9688, -120.8) centre (137.4688, -120.8) ccw
  line L340 (77.9688, -108.3) -> (83.9688, -108.3)
  line L341 (77.9688, -123.3) -> (83.9688, -123.3)
  line L342 (77.4688, -108.8) -> (77.4688, -122.8)
  line L343 (84.4688, -108.8) -> (84.4688, -122.8)
  arc A340 (77.9688, -108.3) -> (77.4688, -108.8) centre (77.9688, -108.8) ccw
  arc A341 (84.4688, -108.8) -> (83.9688, -108.3) centre (83.9688, -108.8) ccw
  arc A342 (77.4688, -122.8) -> (77.9688, -123.3) centre (77.9688, -122.8) ccw
  arc A343 (83.9688, -123.3) -> (84.4688, -122.8) centre (83.9688, -122.8) ccw
  line L344 (177.9688, -108.3) -> (183.9688, -108.3)
  line L345 (177.9688, -123.3) -> (183.9688, -123.3)
  line L346 (177.4688, -108.8) -> (177.4688, -122.8)
  line L347 (184.4688, -108.8) -> (184.4688, -122.8)
  arc A344 (177.9688, -108.3) -> (177.4688, -108.8) centre (177.9688, -108.8) ccw
  arc A345 (184.4688, -108.8) -> (183.9688, -108.3) centre (183.9688, -108.8) ccw
  arc A346 (177.4688, -122.8) -> (177.9688, -123.3) centre (177.9688, -122.8) ccw
  arc A347 (183.9688, -123.3) -> (184.4688, -122.8) centre (183.9688, -122.8) ccw
  line L348 (195.9063, -107.3) -> (208.9062, -107.3)
  line L349 (195.9063, -121.3) -> (208.9062, -121.3)
  line L350 (195.4063, -107.8) -> (195.4063, -120.8)
  line L351 (209.4062, -107.8) -> (209.4062, -120.8)
  arc A348 (195.9063, -107.3) -> (195.4063, -107.8) centre (195.9063, -107.8) ccw
  arc A349 (209.4062, -107.8) -> (208.9062, -107.3) centre (208.9062, -107.8) ccw
  arc A350 (195.4063, -120.8) -> (195.9063, -121.3) centre (195.9063, -120.8) ccw
  arc A351 (208.9062, -121.3) -> (209.4062, -120.8) centre (208.9062, -120.8) ccw
  line L352 (219.7188, -107.3) -> (232.7188, -107.3)
  line L353 (219.7188, -121.3) -> (232.7188, -121.3)
  line L354 (219.2188, -107.8) -> (219.2188, -120.8)
  line L355 (233.2188, -107.8) -> (233.2188, -120.8)
  arc A352 (219.7188, -107.3) -> (219.2188, -107.8) centre (219.7188, -107.8) ccw
  arc A353 (233.2188, -107.8) -> (232.7188, -107.3) centre (232.7188, -107.8) ccw
  arc A354 (219.2188, -120.8) -> (219.7188, -121.3) centre (219.7188, -120.8) ccw
  arc A355 (232.7188, -121.3) -> (233.2188, -120.8) centre (232.7188, -120.8) ccw
  line L356 (243.5313, -107.3) -> (256.5312, -107.3)
  line L357 (243.5313, -121.3) -> (256.5312, -121.3)
  line L358 (243.0312, -107.8) -> (243.0312, -120.8)
  line L359 (257.0312, -107.8) -> (257.0312, -120.8)
  arc A356 (243.5313, -107.3) -> (243.0312, -107.8) centre (243.5313, -107.8) ccw
  arc A357 (257.0312, -107.8) -> (256.5312, -107.3) centre (256.5312, -107.8) ccw
  arc A358 (243.0312, -120.8) -> (243.5313, -121.3) centre (243.5313, -120.8) ccw
  arc A359 (256.5312, -121.3) -> (257.0312, -120.8) centre (256.5312, -120.8) ccw
  line L360 (267.3438, -107.3) -> (280.3438, -107.3)
  line L361 (267.3438, -121.3) -> (280.3438, -121.3)
  line L362 (266.8438, -107.8) -> (266.8438, -120.8)
  line L363 (280.8438, -107.8) -> (280.8438, -120.8)
  arc A360 (267.3438, -107.3) -> (266.8438, -107.8) centre (267.3438, -107.8) ccw
  arc A361 (280.8438, -107.8) -> (280.3438, -107.3) centre (280.3438, -107.8) ccw
  arc A362 (266.8438, -120.8) -> (267.3438, -121.3) centre (267.3438, -120.8) ccw
  arc A363 (280.3438, -121.3) -> (280.8438, -120.8) centre (280.3438, -120.8) ccw
  line L364 (293.5375, -107.3) -> (306.5375, -107.3)
  line L365 (293.5375, -121.3) -> (306.5375, -121.3)
  line L366 (293.0375, -107.8) -> (293.0375, -120.8)
  line L367 (307.0375, -107.8) -> (307.0375, -120.8)
  arc A364 (293.5375, -107.3) -> (293.0375, -107.8) centre (293.5375, -107.8) ccw
  arc A365 (307.0375, -107.8) -> (306.5375, -107.3) centre (306.5375, -107.8) ccw
  arc A366 (293.0375, -120.8) -> (293.5375, -121.3) centre (293.5375, -120.8) ccw
  arc A367 (306.5375, -121.3) -> (307.0375, -120.8) centre (306.5375, -120.8) ccw
  line L368 (312.5875, -107.3) -> (325.5875, -107.3)
  line L369 (312.5875, -121.3) -> (325.5875, -121.3)
  line L370 (312.0875, -107.8) -> (312.0875, -120.8)
  line L371 (326.0875, -107.8) -> (326.0875, -120.8)
  arc A368 (312.5875, -107.3) -> (312.0875, -107.8) centre (312.5875, -107.8) ccw
  arc A369 (326.0875, -107.8) -> (325.5875, -107.3) centre (325.5875, -107.8) ccw
  arc A370 (312.0875, -120.8) -> (312.5875, -121.3) centre (312.5875, -120.8) ccw
  arc A371 (325.5875, -121.3) -> (326.0875, -120.8) centre (325.5875, -120.8) ccw
  line L372 (331.6375, -107.3) -> (344.6375, -107.3)
  line L373 (331.6375, -121.3) -> (344.6375, -121.3)
  line L374 (331.1375, -107.8) -> (331.1375, -120.8)
  line L375 (345.1375, -107.8) -> (345.1375, -120.8)
  arc A372 (331.6375, -107.3) -> (331.1375, -107.8) centre (331.6375, -107.8) ccw
  arc A373 (345.1375, -107.8) -> (344.6375, -107.3) centre (344.6375, -107.8) ccw
  arc A374 (331.1375, -120.8) -> (331.6375, -121.3) centre (331.6375, -120.8) ccw
  arc A375 (344.6375, -121.3) -> (345.1375, -120.8) centre (344.6375, -120.8) ccw
  line L376 (0, -123.825) -> (347.6625, -123.825)
  line L377 (0, -4.7625) -> (347.6625, -4.7625)
  line L378 (0, -123.825) -> (0, -4.7625)
  line L379 (347.6625, -123.825) -> (347.6625, -4.7625)
  point P0 (165.5613, -65.3602)